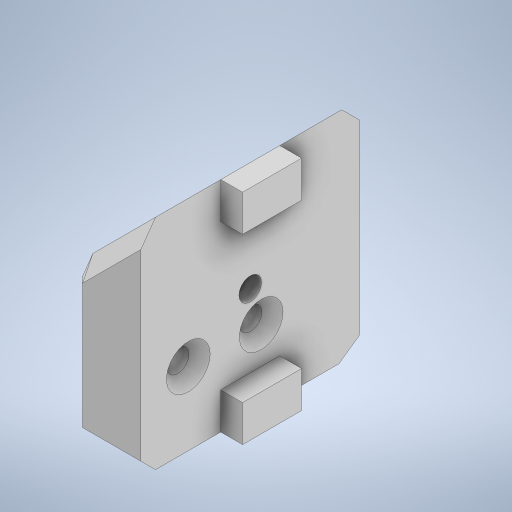
# Autodesk Inventor part: 电源支架
Saved by Autodesk Inventor 2023 (Build 270158000, 158)
## iProperties
Created: 2022-04-22
Part Number: 电源支架
Material: 常规
Document SubType Name: Modeling
Designer: Zhong
Density: 1 g/cm^3
Appearance: 默认
Author: Zhong
Autodesk Inventor part; units mm, degrees
ref_plane "XZ Plane" through (0, 0, 0) normal (0, 1, 0) x (-1, 0, 0)
ref_plane "XY Plane" through (0, 0, 0) normal (0, 0, 1) x (1, 0, 0)
sketch "草图1" plane through (0, 0, 0) normal (1, 0, 0) x (0, 1, 0)
  line L0 (0, 0) -> (20, 0)
  line L1 (20, 0) -> (20, -40)
  line L2 (20, -40) -> (0, -40)
  line L3 (0, -40) -> (0, 0)
  dimension "d0" = 20
  dimension "d1" = 40
  constraints: 8 end point, 2 parallel, 1 horizontal, 1 perpendicular
  measures "d0" distance of L1.end L2.end
  measures "d1" distance of L2.end L0.start
ref_plane "工作平面1" through (10, 0, 0) normal (1, 0, 0) x (0, 1, 0)
sketch "草图2" plane through (10, 0, 0) normal (1, 0, 0) x (0, 1, 0)
  line L0 (0, 0) -> (30, 0)
  line L1 (30, 0) -> (30, -30)
  line L2 (30, -30) -> (0, -30)
  line L3 (0, -30) -> (0, 0)
  dimension "d7" = 30
  dimension "d8" = 30
  constraints: 8 end point, 2 parallel, 1 horizontal, 1 perpendicular
  measures "d7" distance of L1.end L2.end
  measures "d8" distance of L0.end L1.end
loft "放样1" add profiles "草图2", "草图1"
sketch "草图3" plane through (10, 0, 0) normal (1, 0, 0) x (0, 0, -1)
  line L0 (0, 0) -> (0, 30) projected
  line L1 (30, 0) -> (0, 0) projected
  point P0 (6.5, 10)
  point P1 (16.5, 10)
  dimension "d14" = 10
  dimension "d15" = 6.5
  dimension "d16" = 10
  constraints: 1 horizontal alignment
  measures "d14" distance of point (16.5, 10) point (6.5, 10)
  measures "d15" distance from line of L0 point (6.5, 10)
  measures "d16" distance from line of L1 point (6.5, 10)
hole "孔1" at (10, 10, -6.5) at (10, 10, -16.5) direction (-1, 0, 0) diameter 3.1 end through all countersink diameter 6 countersink angle 90
sketch "草图5" plane through (0, 0, 0) normal (-1, 0, 0) x (0, 0, 1)
  line L0 (0, 0) -> (0, 20) projected
  point P0 (-15, 15)
  dimension "d26" = 15
  dimension "d27" = 15
  measures "d26" horizontal distance of L0.start point (-15, 15)
  measures "d27" distance from line of L0 point (-15, 15)
hole "孔2" at (0, 15, -15) direction (1, 0, 0) diameter 3.1 end through all countersink diameter 6 countersink angle 90
sketch "草图6" plane through (10, 0, 0) normal (1, 0, 0) x (0, 0, -1)
  line L0 (0, 30) -> (30, 30) projected
  line L1 (10.95, 30) -> (19.05, 30)
  line L2 (19.05, 30) -> (19.05, 25)
  line L3 (19.05, 25) -> (10.95, 25)
  line L4 (10.95, 25) -> (10.95, 30)
  line L5 (30, 0) -> (0, 0) projected
  line L6 (10.95, 5) -> (19.05, 5)
  line L7 (19.05, 5) -> (19.05, 0)
  line L8 (19.05, 0) -> (10.95, 0)
  line L9 (10.95, 0) -> (10.95, 5)
  line L10 (0, 0) -> (0, 30) projected
  point P0 (15, 30)
  dimension "d35" = 8.1
  dimension "d36" = 5
  dimension "d37" = 15
  constraints: 16 end point, 4 parallel, 4 point on line, 2 horizontal, 2 perpendicular, 1 collinear, 1 midpoint
  measures "d35" distance of L2.end L3.end
  measures "d36" distance of L1.end L2.end
  measures "d37" distance from line of L10 point (15, 30)
extrude "拉伸1" add sketch "草图6" along normal blind 3
chamfer "倒角1" distance 2 angle 45 8 edges at (5, 25, 0) (5, 25, -35) (5, 0, -35) (0, 10, -40) (0, 0, -20) (5, 0, 0) (0, 20, -20) (0, 10, 0)
